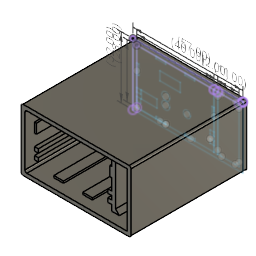
DD-boitier-V4 (Autodesk Fusion 360 design; units mm, degrees)
part number: 2025-12-19-14-32-53-043
Autodesk Fusion 360 part; units mm, degrees
sketch "Esquisse1" plane through (0, 0, 0) normal (0, 1, 0) x (1, 0, 0)
  line L0 (0, -28) -> (40, -28)
  line L1 (40, -28) -> (40, 0)
  line L2 (40, 0) -> (42, 0)
  line L3 (42, 0) -> (42, -28)
  line L4 (42, -28) -> (40, -28)
  line L5 (40, -28) -> (40, 0)
  line L6 (42, 0) -> (53, 0)
  line L7 (53, 0) -> (53, -28)
  line L8 (53, -28) -> (42, -28)
  line L9 (42, -28) -> (42, 0)
  line L10 (12, 0) -> (15, 0)
  line L11 (25, 0) -> (28, 0)
  line L12 (10, -28) -> (15, -28)
  line L13 (15, -28) -> (15, -27)
  line L14 (15, -27) -> (10, -27)
  line L15 (10, -27) -> (10, -28)
  line L16 (30, -28) -> (25, -28)
  line L17 (25, -28) -> (25, -27)
  line L18 (25, -27) -> (30, -27)
  line L19 (30, -27) -> (30, -28)
  line L20 (0, -3) -> (2, -3)
  line L21 (2, -3) -> (2, -5)
  line L22 (2, -5) -> (0, -5)
  line L23 (0, -5) -> (0, -3)
  line L24 (40, -3) -> (38, -3)
  line L25 (38, -3) -> (38, -5)
  line L26 (38, -5) -> (40, -5)
  line L27 (40, -5) -> (40, -3)
  line L28 (40, -7) -> (38, -7)
  line L29 (38, -7) -> (38, -9)
  line L30 (38, -9) -> (40, -9)
  line L31 (40, -9) -> (40, -7)
  line L32 (2.4548, -4.9937) -> (10.4548, -4.9937)
  line L33 (10.4548, -4.9937) -> (10.4548, -9.0296)
  line L34 (10.4548, -9.0296) -> (2.4548, -9.0296)
  line L35 (2.4548, -9.0296) -> (2.4548, -4.9937)
  circle A0 centre (26, -10) radius 1.75
  circle A1 centre (15, -8.5) radius 2
  circle A2 centre (15, -12.5) radius 2
  line L36 (0, 0) -> (40, 0)
  line L37 (0, 0) -> (0, -28)
  line L38 (0, -7) -> (2, -7)
  line L39 (2, -7) -> (2, -9)
  line L40 (2, -9) -> (0, -9)
  line L41 (0, -9) -> (0, -7)
  line L42 (-2, -30) -> (55, -30)
  line L43 (55, -30) -> (55, 2)
  line L44 (55, 2) -> (-2, 2)
  line L45 (-2, 2) -> (-2, -30)
  line L46 (0, 0) -> (15, 0)
  line L47 (0, -16.5) -> (0, 0)
  line L48 (12, -18) -> (22.5073, -18)
  line L49 (22.5073, -18) -> (22.5073, -22.5)
  line L50 (22.5073, -22.5) -> (12, -22.5)
  line L51 (12, -22.5) -> (12, -18)
  line L52 (0, -20) -> (1, -20)
  line L53 (1, -20) -> (1, -15)
  line L54 (1, -15) -> (0, -15)
  line L55 (0, -15) -> (0, -20)
  line L56 (40, -16) -> (40, -20)
  line L57 (44, -28) -> (42, -26)
  line L58 (51, -28) -> (53, -26)
  line L59 (53, -2) -> (51, 0)
  line L60 (44, 0) -> (42, -2)
  line L61 (10, 0) -> (15, 0)
  line L62 (15, 0) -> (15, -1)
  line L63 (15, -1) -> (10, -1)
  line L64 (10, -1) -> (10, 0)
  line L65 (25, 0) -> (30, 0)
  line L66 (30, 0) -> (30, -1)
  line L67 (30, -1) -> (25, -1)
  line L68 (25, -1) -> (25, 0)
  line L69 (40, -20) -> (39, -20)
  line L70 (39, -20) -> (39, -15)
  line L71 (39, -15) -> (40, -15)
  line L72 (40, -15) -> (40, -20)
  dimension "d42" = 28
  dimension "d43" = 32
  dimension "d44" = 40
  dimension "d45" = 2
  dimension "d46" = 11
  dimension "d47" = 57
  constraint horizontal L0
  constraint vertical L1
  constraint horizontal L2
  constraint vertical L3
  constraint horizontal L4
  constraint vertical L5
  constraint horizontal L6
  constraint vertical L7
  constraint horizontal L8
  constraint vertical L9
  constraint horizontal L10
  constraint horizontal L11
  constraint horizontal L12
  constraint vertical L13
  constraint horizontal L14
  constraint vertical L15
  constraint horizontal L16
  constraint vertical L17
  constraint horizontal L18
  constraint vertical L19
  constraint horizontal L20
  constraint vertical L21
  constraint horizontal L22
  constraint vertical L23
  constraint horizontal L24
  constraint vertical L25
  constraint horizontal L26
  constraint vertical L27
  constraint horizontal L28
  constraint vertical L29
  constraint horizontal L30
  constraint vertical L31
  constraint horizontal L32
  constraint vertical L33
  constraint horizontal L34
  constraint vertical L35
  constraint perpendicular L1 L36
  constraint perpendicular L0 L37
  constraint horizontal L38
  constraint vertical L39
  constraint horizontal L40
  constraint vertical L41
  constraint horizontal L42
  constraint vertical L43
  constraint horizontal L44
  constraint vertical L45
  constraint horizontal L46
  constraint vertical L47
  constraint horizontal L48
  constraint vertical L49
  constraint horizontal L50
  constraint vertical L51
  constraint horizontal L52
  constraint vertical L53
  constraint horizontal L54
  constraint vertical L55
  constraint vertical L56
  constraint perpendicular L57 L58
  constraint perpendicular L58 L59
  constraint perpendicular L59 L60
  constraint horizontal L61
  constraint vertical L62
  constraint horizontal L63
  constraint vertical L64
  constraint horizontal L65
  constraint vertical L66
  constraint horizontal L67
  constraint vertical L68
  constraint horizontal L69
  constraint vertical L70
  constraint horizontal L71
  constraint vertical L72
  measures "d42" distance of L0.start L36.start
  measures "d43" distance of L42.start L44.end
  measures "d44" distance of L1.end L36.start
  measures "d45" distance of L1.end L2.end
  measures "d46" distance of L2.end L6.end
  measures "d47" distance of L43.end L44.end
sketch "Esquisse2" plane through (0, 0, 0) normal (0, 1, 0) x (1, 0, 0)
sketch "Esquisse3" plane through (0, 0, 0) normal (0, 1, 0) x (1, 0, 0)
  line L0 (-2, -30) -> (55, -30)
  line L1 (-2, 2) -> (-2, -30)
  dimension "d54" = 57
  dimension "d55" = 32
  measures "d54" distance of L0.start L0.end
  measures "d55" distance of L0.start L1.start
extrude "Extrusion11" add sketch "Esquisse1" along normal blind 2 contours L0 L1 L5 L13 L14 L15 L17 L18 L19 L20 L21 L22 L24 L25 L26 L28 L29 L30 L36 L37 L38 L39 L40 L46 L47 L52 L53 L54 L62 L63 L64 L66 L67 L68 L69 L70 L71 | L0 L12 L13 L14 L15 | L37 L47 L52 L53 L54 L55 | L0 L16 L17 L18 L19 | L37 L38 L39 L40 L41 L47 | L1 L2 L3 L4 L5 L9 L27 L31 L56 L72 | L1 L5 L56 L69 L70 L71 L72 | L3 L8 L9 L57 | L20 L21 L22 L23 L37 L47 | L3 L6 L7 L8 L9 L57 L58 L59 L60 | L3 L6 L9 L60 | L7 L8 L58 | L1 L5 L28 L29 L30 L31 | L10 L36 L46 L61 L62 L63 L64 | L6 L7 L59 | L1 L5 L24 L25 L26 L27 | L11 L36 L65 L66 L67 L68 | L42 L43 L44 L45 makes body 1
extrude "Extrusion12" add sketch "Esquisse1" against normal blind 53 separate body contours L0 L12 L13 L14 L15 | L37 L47 L52 L53 L54 L55 | L0 L16 L17 L18 L19 | L37 L38 L39 L40 L41 L47 | L1 L2 L3 L4 L5 L9 L27 L31 L56 L72 | L1 L5 L56 L69 L70 L71 L72 | L3 L8 L9 L57 | L20 L21 L22 L23 L37 L47 | L3 L6 L9 L60 | L7 L8 L58 | L1 L5 L28 L29 L30 L31 | L10 L36 L46 L61 L62 L63 L64 | L6 L7 L59 | L1 L5 L24 L25 L26 L27 | L11 L36 L65 L66 L67 L68 makes body 2 at (26.6667, -17.6667, 27) makes body 3 at (0, -17.6667, 4.3333) makes body 4 at (13.3333, -17.6667, 27) makes body 5 at (11.6667, -17.6667, 0) makes body 6 at (51.6667, -35.3333, 27.3333) makes body 7 at (42, -35.3333, 18) makes body 8 at (0, -17.6667, 7.6667) makes body 9 at (0, -17.6667, 16.6667) makes body 10 at (28.3333, -17.6667, 1) makes body 11 at (52.3333, -17.6667, 1.3333)
extrude "Extrusion13" add sketch "Esquisse1" against normal blind 58 contours L42 L43 L44 L45 bodies 2 3 4 5 6 7 8 9 10 11
fillet "Congé1" radius 1 6 edges at (-2, -29, 30) (55, -29, 30) (0, -29, 28) (0, -29, 0) (-2, -29, -2) (55, -29, -2) on bodies 2
sketch "Esquisse4" plane through (0, 0, 0) normal (0, 0, 1) x (1, 0, 0)
fillet "Congé2" radius 1 1 edges at (55, 1, -2) on bodies 1
fillet "Congé3" radius 1 1 edges at (-2, 1, -2) on bodies 1
fillet "Congé4" radius 1 1 edges at (55, 1, 30) on bodies 1
fillet "Congé5" radius 1 1 edges at (-2, 1, 30) on bodies 1
sketch "Esquisse5" plane through (0, 0, 0) normal (0, 1, 0) x (1, 0, 0)
  line L0 (-2, 2) -> (-2, -30)
  line L1 (0, 0) -> (0, -28)
  line L2 (-2, -30) -> (55, -30)
  line L3 (0, -28) -> (40, -28)
  line L4 (42, -28) -> (40, -28)
  line L5 (53, -28) -> (42, -28)
  dimension "d80" = 32
  dimension "d81" = 28
  dimension "d82" = 57
  dimension "d83" = 40
  dimension "d84" = 2
  dimension "d85" = 11
  measures "d80" distance of L0.start L0.end
  measures "d81" distance of L1.start L1.end
  measures "d82" distance of L0.end L2.end
  measures "d83" distance of L1.end L3.end
  measures "d84" distance of L4.start L3.end
  measures "d85" distance of L5.start L4.start
extrude "Extrusion1" [suppressed]
extrude "Extrusion2" [suppressed]
extrude "Extrusion3" [suppressed]
